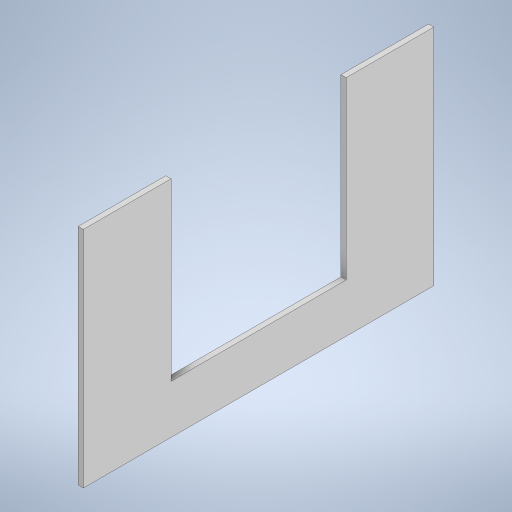
# Autodesk Inventor part: WI-CoverRS3
Saved by Autodesk Inventor 2024.3 (Build 283343000, 343)
## iProperties
Created: 2025-06-13
Part Number: WI-CoverRS3
Material: Generic
Document SubType Name: Modeling
Designer: ajclo
Density: 1 g/cm^3
Appearance: Default
Author: ajclo
Autodesk Inventor part; units mm, degrees
ref_plane "YZ Plane" through (0, 0, 0) normal (1, 0, 0) x (0, 1, 0)
ref_plane "XZ Plane" through (0, 0, 0) normal (0, 1, 0) x (-1, 0, 0)
ref_plane "XY Plane" through (0, 0, 0) normal (0, 0, 1) x (1, 0, 0)
sketch "Sketch1" plane through (0, 0, 0) normal (1, 0, 0) x (0, 1, 0)
  line L0 (-63.921, 100) -> (63.921, 100)
  line L1 (63.921, 100) -> (63.921, -100)
  line L2 (63.921, -100) -> (-63.921, -100)
  line L3 (-63.921, -100) -> (-63.921, 100)
  line L4 (-63.921, 100) -> (63.921, -100) construction
  line L5 (63.921, 100) -> (-63.921, -100) construction
  line L6 (63.921, 50) -> (-36.079, 50)
  line L7 (-36.079, 50) -> (-36.079, -50)
  line L8 (-36.079, -50) -> (63.921, -50)
  line L9 (63.921, -50) -> (63.921, 50)
  point P0 (0, 0)
  point P1 (63.921, -50)
  dimension "d0" = 200
  dimension "d1" = 127.842
  dimension "d2" = 100
  dimension "d3" = 100
  dimension "d4" = 50
  constraints: 20 end point, 4 parallel, 2 horizontal, 2 midpoint, 2 perpendicular, 1 point on line
  measures "d0" distance of L0.end L1.end
  measures "d1" distance of L1.end L2.end
  measures "d2" distance of L6.end L7.end
  measures "d3" distance of L7.end L8.end
  measures "d4" distance between parallel lines of L2 L8
extrude "Extrusion1" add sketch "Sketch1" along normal blind 3 contours L0 L1 L6 L7 L8 L2 L3
equation "\"d3\" = d2"
body "Solid1"
